Autodesk Fusion 360 part; units mm, degrees
(part 2 of 2)
  constraint tangent L241 A239
  constraint tangent L240 A239
  constraint tangent L231 A240
  constraint tangent L232 A240
  constraint tangent L230 A241
  constraint tangent L231 A241
  constraint tangent L229 A242
  constraint tangent L230 A242
  constraint tangent L228 A243
  constraint tangent L229 A243
  constraint tangent L227 A244
  constraint tangent L228 A244
  constraint tangent L226 A245
  constraint tangent L227 A245
  constraint tangent L226 A246
  constraint tangent L245 A246
  constraint tangent L244 A247
  constraint tangent L245 A247
  constraint tangent L244 A248
  constraint tangent L243 A248
  constraint tangent L242 A249
  constraint tangent L243 A249
  constraint tangent L246 A250
  constraint tangent L240 A250
  constraint tangent L239 A251
  constraint tangent L246 A251
  constraint tangent L247 A252
  constraint tangent L239 A252
  constraint tangent L238 A253
  constraint tangent L247 A253
  constraint tangent L238 A254
  constraint tangent L237 A254
  constraint tangent L237 A255
  constraint tangent L236 A255
  constraint tangent L236 A256
  constraint tangent L235 A256
  constraint tangent L235 A257
  constraint tangent L234 A257
  constraint perpendicular L249 L253
  constraint collinear L251 L252
  constraint collinear L253 L254
  constraint tangent L249 A258
  constraint tangent L251 A258
  constraint tangent L249 A259
  constraint tangent L254 A259
  constraint tangent L250 A260
  constraint tangent L252 A260
  constraint tangent L250 A261
  constraint tangent L253 A261
  constraint concentric A3 A262
  constraint concentric A4 A263
  constraint concentric A0 A264
  constraint concentric A1 A265
  constraint concentric A111 A266
  constraint concentric A112 A267
  constraint vertical L248
  constraint tangent L255 A268
  constraint tangent L256 A268
  constraint tangent L255 A269
  constraint tangent L256 A270
  constraint coincident L213 L257.end
  constraint tangent L248 A271
  constraint coincident L257.start A271.start
  constraint tangent L248 A272
  measures "d1" diameter of A0
  measures "d2" diameter of A1
  measures "d3" diameter of A2
  measures "d4" diameter of A3
  measures "d5" diameter of A4
  measures "d9" diameter of A111
  measures "d12" diameter of A112
  measures "d367" diameter of A262
  measures "d368" diameter of A263
  measures "d369" diameter of A264
  measures "d370" diameter of A265
  measures "d393" diameter of A266
  measures "d394" diameter of A267
extrude "Extrude1" add sketch "mriya" along normal blind 10.5 contours L178 L179 L204 A214 L205 A215 L206 A216 L207 A217 L208 A218 L209 A219 L210 A220 L211 A221 L212 A222 L213 L214 A224 L215 A225 L216 A226 L217 A227 L218 A228 L219 A229 L220 A230 L221 A231 L222 A232 L223 A233 L224 A234 L225 A235 L226 L227 L228 L229 L230 L231 L232 L233 L234 L235 L236 L237 L238 L239 L240 L241 L242 L243 L244 L245 L246 L247 A236 A237 A239 A240 A241 A242 A243 A244 A245 A246 A247 A248 A249 A250 A251 A252 A253 A254 A255 A256 A257 L257 makes body 1
extrude "Extrude2" add sketch "mriya" along normal blind 17 contours L178 L179 L213 A223 L214 L241 L242 A238 bodies 1
extrude "Extrude3" add sketch "mriya" along normal blind 3.7 contours A114 | A115 | A116 | A117 | L204 A214 L205 A215 L206 A216 L207 A217 L208 A218 L209 A219 L210 A220 L211 A221 L212 A222 L213 L214 A224 L215 A225 L216 A226 L217 A227 L218 A228 L219 A229 L220 A230 L221 A231 L222 A232 L223 A233 L224 A234 L225 A235 L248 L255 L256 A268 A269 A270 L257 A271 A272 | L213 A223 L214 L255 L256 A268 A269 A270 | L213 L248 A271 A272 | A266 | A267 bodies 1
extrude "Extrude13" add sketch "mriya" along normal blind 1.8 contours A2 | L108 L109 A118 A119 A120 L186 L187 L190 A198 A199 | A121 L110 A122 L111 A123 L180 L181 L184 A202 A203 | A124 L112 A125 L113 A126 L114 A127 L115 | A128 L116 A129 L117 A130 L118 A131 L119 | A132 L120 A133 A134 L121 L188 L189 L191 A200 A201 | A135 L122 A136 A137 L123 L182 L183 L185 A204 A205 | A138 L124 A139 L125 A140 L126 A141 L127 | A142 L128 A143 L129 A144 L130 A145 L131 | A146 L132 A147 L133 A148 L134 A149 L135 | A150 L136 A151 L137 A152 L138 A153 L139 | A154 L140 A155 L141 A156 L142 A157 L143 | A158 L144 A159 L145 A160 L146 A161 L147 | A162 L148 A163 L149 A164 L150 A165 L151 | A166 L152 A167 L153 A168 L194 L195 L196 A206 A207 | A169 L154 A170 L155 A171 L156 A172 L157 | A173 L158 A174 L159 A175 L200 L201 L202 A210 A211 | A176 L160 A177 L161 A178 L162 A179 L163 | A180 A181 L164 A182 L165 L198 L199 L203 A212 A213 | A183 L166 A184 L167 A185 L168 A186 L169 | A187 A188 L170 A189 L171 L192 L193 L197 A208 A209 | A190 L172 A191 L173 A192 L174 A193 L175 | A194 L176 A195 L249 L251 L254 A258 A259 | A196 L177 A197 L250 L252 L253 A260 A261 bodies 1
extrude "Extrude14" add sketch "mriya" along normal blind 2.2 contours A0 | A1 | A3 | A4 bodies 1
extrude "Extrude6" add sketch "mriya" along normal blind 1 from surface at 14.3 contours L213 A223 L214 L255 L256 A268 A269 A270 bodies 1
extrude "Extrude12" add sketch "mriya" along normal blind 1 from surface at 7.7 contours L213 L248 A271 A272 bodies 1
sketch "power switch" plane through (-4.4, 0, 0) normal (1, 0, 0) x (0, 1, 0)
  line L0 (1.7932, 0) -> (76.6932, 0)
  line L1 (76.6932, 0) -> (76.6932, 17)
  line L2 (76.6932, 17) -> (19.2932, 17)
  line L3 (19.2932, 17) -> (19.2932, 10.5)
  line L4 (19.2932, 10.5) -> (1.7932, 10.5)
  line L5 (1.7932, 10.5) -> (1.7932, 0)
  line L6 (24.0932, 4.15) -> (24.0932, 9.1)
  line L7 (37.2932, 3.75) -> (24.4932, 3.75)
  arc A0 (37.6932, 9.1) -> (37.2932, 9.5) centre (37.2932, 9.1) ccw
  line L8 (36.0932, 8.1) -> (36.0932, 5.15)
  line L9 (25.6932, 8.1) -> (36.0932, 8.1)
  line L10 (36.0932, 5.15) -> (25.6932, 5.15)
  line L11 (25.6932, 5.15) -> (25.6932, 8.1)
  line L12 (24.4932, 9.5) -> (37.2932, 9.5)
  arc A1 (24.0932, 4.15) -> (24.4932, 3.75) centre (24.4932, 4.15) ccw
  arc A2 (37.2932, 3.75) -> (37.6932, 4.15) centre (37.2932, 4.15) ccw
  line L13 (37.6932, 9.1) -> (37.6932, 4.15)
  arc A3 (24.4932, 9.5) -> (24.0932, 9.1) centre (24.4932, 9.1) ccw
  constraint perpendicular L10 L11
  constraint vertical L11
  constraint perpendicular L9 L11
  constraint vertical L8
  constraint tangent A0 L12
  constraint tangent A0 L13
  constraint tangent A2 L13
  constraint tangent L7 A2
  constraint tangent L7 A1
  constraint tangent L6 A1
  constraint tangent L6 A3
  constraint tangent L12 A3
extrude "Extrude8" cut sketch "power switch" against normal blind 2.5 contours L8 L9 L10 L11 bodies 1
extrude "Extrude9" cut sketch "power switch" against normal blind 1 contours L6 L7 A0 L12 A1 A2 L13 A3 bodies 1
chamfer "Chamfer13" distance 1.19 angle 40 8 edges at (-4.4, 30.8932, 3.75) (-4.4, 24.2104, 3.8672) (-4.4, 24.0932, 6.625) (-4.4, 24.2104, 9.3828) (-4.4, 30.8932, 9.5) (-4.4, 37.576, 9.3828) (-4.4, 37.6932, 6.625) (-4.4, 37.576, 3.8672) measured on face at (-4.4, 63.6932, 8.7) measured on face at (-4.4, 63.6932, 8.7) measured on face at (-4.4, 63.6932, 8.7) measured on face at (-4.4, 63.6932, 8.7) measured on face at (-4.4, 63.6932, 8.7) measured on face at (-4.4, 63.6932, 8.7) measured on face at (-4.4, 63.6932, 8.7) measured on face at (-4.4, 63.6932, 8.7) on bodies 1
chamfer "Chamfer14" distance 0.8 angle 45 4 edges at (-6.9, 30.8932, 5.15) (-6.9, 25.6932, 6.625) (-6.9, 30.8932, 8.1) (-6.9, 36.0932, 6.625) on bodies 1
sketch "usb-c" plane through (0, 80.6932, 0) normal (0, 1, 0) x (-1, 0, 0)
  line L0 (8.4, 0) -> (41.0674, 0)
  line L1 (41.0674, 0) -> (41.0674, 10.5)
  line L2 (41.0674, 10.5) -> (25.8, 10.5)
  line L3 (25.8, 10.5) -> (25.8, 17)
  line L4 (25.8, 17) -> (8.4, 17)
  line L5 (8.4, 17) -> (8.4, 0)
  line L6 (19.7003, 8.8) -> (13.1003, 8.8)
  line L7 (21.9003, 12.8) -> (21.9003, 8.4)
  line L8 (21.1002, 11) -> (21.1002, 10.2)
  arc A0 (11.3003, 13.2) -> (10.9002, 12.8) centre (11.3003, 12.8) ccw
  arc A1 (21.5003, 8) -> (21.9002, 8.4) centre (21.5003, 8.4) ccw
  arc A2 (19.7003, 8.8) -> (21.1003, 10.2) centre (19.7003, 10.2) ccw
  line L9 (11.7003, 10.2) -> (11.7003, 11)
  line L10 (21.5003, 8) -> (11.3002, 8)
  arc A3 (21.1002, 11) -> (19.7003, 12.4) centre (19.7003, 11) ccw
  arc A4 (13.1002, 12.4) -> (11.7002, 11) centre (13.1002, 11) ccw
  line L11 (11.3003, 13.2) -> (21.5003, 13.2)
  line L12 (13.1002, 12.4) -> (19.7003, 12.4)
  arc A5 (21.9002, 12.8) -> (21.5003, 13.2) centre (21.5003, 12.8) ccw
  arc A6 (10.9002, 8.4) -> (11.3002, 8) centre (11.3002, 8.4) ccw
  line L13 (10.9002, 8.4) -> (10.9002, 12.8)
  arc A7 (11.7003, 10.2) -> (13.1003, 8.8) centre (13.1003, 10.2) ccw
  constraint tangent L9 A4
  constraint tangent A4 L12
  constraint tangent A3 L12
  constraint tangent L8 A3
  constraint tangent L6 A2
  constraint tangent L8 A2
  constraint tangent L6 A7
  constraint tangent L9 A7
  constraint perpendicular L7 L11
  constraint perpendicular L10 L13
  constraint horizontal L10
  constraint perpendicular L7 L10
  constraint tangent A0 L11
  constraint tangent A0 L13
  constraint tangent L11 A5
  constraint tangent L7 A5
  constraint tangent A6 L13
  constraint tangent L10 A6
  constraint tangent A1 L10
  constraint tangent L7 A1
extrude "Extrude17" cut sketch "usb-c" against normal blind 2.5 contours L6 L8 A2 L9 A3 A4 L12 A7 bodies 1
extrude "Extrude18" cut sketch "usb-c" against normal blind 1 contours L7 A0 A1 L10 L11 A5 A6 L13 bodies 1
chamfer "Chamfer23" distance 1.19 angle 40 8 edges at (-16.4003, 80.6932, 8) (-11.0174, 80.6932, 8.1172) (-10.9003, 80.6932, 10.6) (-11.0174, 80.6932, 13.0828) (-16.4003, 80.6932, 13.2) (-21.7831, 80.6932, 13.0828) (-21.9003, 80.6932, 10.6) (-21.7831, 80.6932, 8.1172) measured on face at (-23.679, 80.6932, 2.6687) measured on face at (-23.679, 80.6932, 2.6687) measured on face at (-23.679, 80.6932, 2.6687) measured on face at (-23.679, 80.6932, 2.6687) measured on face at (-23.679, 80.6932, 2.6687) measured on face at (-23.679, 80.6932, 2.6687) measured on face at (-23.679, 80.6932, 2.6687) measured on face at (-23.679, 80.6932, 2.6687) on bodies 1
chamfer "Chamfer21" distance 0.599 angle 45 3 edges at (-14.85, 78.1932, 14.3) (-7.3979, 77.6953, 14.3) (-6.9, 57.7432, 14.3) on bodies 1
chamfer "Chamfer22" distance 0.6 angle 45 1 edges at (-6.9, 9.5932, 7.7) on bodies 1
chamfer "Chamfer17" distance 1 angle 45 90 edges at (-17.0879, -2.2068, 10.5) (-5.5716, -1.0352, 10.5) (-4.4, 10.5432, 10.5) (-33.4337, 80.6932, 10.5) (-41.4501, 80.7693, 10.5) (-42.3387, 81.5503, 10.5) (-43.8762, 82.7648, 10.5) (-51.4458, 82.9932, 10.5) (-58.2501, 83.0693, 10.5) (-60.2387, 84.9503, 10.5) (-62.8762, 87.2648, 10.5) (-73.4, 87.4932, 10.5) (-83.9238, 87.2648, 10.5) (-86.0613, 85.4503, 10.5) (-87.5499, 84.0693, 10.5) (-94.8542, 83.9932, 10.5) (-102.9238, 83.7648, 10.5) (-107.238, 79.7735, 10.5) (-111.0657, 76.1074, 10.5) (-116.2077, 75.9932, 10.5) (-121.9238, 75.7648, 10.5) (-123.4613, 74.5503, 10.5) (-124.3499, 73.7693, 10.5) (-131.5163, 73.6932, 10.5) (-141.1284, 72.5216, 10.5) (-142.3, 42.8932, 10.5) (-141.1284, 13.2648, 10.5) (-120.4728, 12.0932, 10.5) (-100.9235, 12.4357, 10.5) (-96.4155, 16.4593, 10.5) (-92.7186, 19.941, 10.5) (-84.5898, 20.0932, 10.5) (-75.7143, 19.6842, 10.5) (-70.5474, 11.3702, 10.5) (-65.1972, 2.8703, 10.5) (-56.0828, 2.3932, 10.5) (-48.3499, 2.3171, 10.5) (-47.4613, 1.5361, 10.5) (-45.9238, 0.3216, 10.5) (-37.2542, 0.0932, 10.5) (-29.3499, 0.0171, 10.5) (-28.4613, -0.7639, 10.5) (-26.9238, -1.9784, 10.5) (-17.0879, -2.2068, 0) (-26.9238, -1.9784, 0) (-28.4613, -0.7639, 0) (-29.3499, 0.0171, 0) (-37.2542, 0.0932, 0) (-45.9238, 0.3216, 0) (-47.4613, 1.5361, 0) (-48.3499, 2.3171, 0) (-56.0828, 2.3932, 0) (-65.1972, 2.8703, 0) (-70.5474, 11.3702, 0) (-75.7143, 19.6842, 0) (-84.5898, 20.0932, 0) (-92.7186, 19.941, 0) (-96.4155, 16.4593, 0) (-100.9235, 12.4357, 0) (-120.4728, 12.0932, 0) (-141.1284, 13.2648, 0) (-142.3, 42.8932, 0) (-141.1284, 72.5216, 0) (-131.5163, 73.6932, 0) (-124.3499, 73.7693, 0) (-123.4613, 74.5503, 0) (-121.9238, 75.7648, 0) (-116.2077, 75.9932, 0) (-111.0657, 76.1074, 0) (-107.238, 79.7735, 0) (-102.9238, 83.7648, 0) (-94.8542, 83.9932, 0) (-87.5499, 84.0693, 0) (-86.0613, 85.4503, 0) (-83.9238, 87.2648, 0) (-73.4, 87.4932, 0) (-62.8762, 87.2648, 0) (-60.2387, 84.9503, 0) (-58.2501, 83.0693, 0) (-51.4458, 82.9932, 0) (-43.8762, 82.7648, 0) (-42.3387, 81.5503, 0) (-41.4501, 80.7693, 0) (-24.7337, 80.6932, 0) (-5.5716, 79.5216, 0) (-4.4, 39.2432, 0) (-5.5716, -1.0352, 0) (-4.4, 47.9932, 17) (-5.5716, 79.5216, 17) (-17.1, 80.6932, 17) on bodies 1
fillet "Fillet29" radius 1.2 2 edges at (-4.4, 19.2932, 12.75) (-25.8, 80.6932, 12.75) on bodies 1
chamfer "Chamfer18" distance 1 angle 45 4 edges at (-6.25, 19.2932, 17) (-5.4996, 19.2974, 17) (-25.8, 78.8432, 17) (-25.7958, 79.5936, 17) on bodies 1
chamfer "Chamfer20" distance 0.9 angle 45 6 edges at (-11.1256, 22.891, 0) (-23.6256, 22.891, 0) (-45.9256, 22.941, 0) (-45.9256, 60.941, 0) (-121.9256, 34.941, 0) (-121.9256, 53.941, 0) on bodies 1
sketch "silicone feets" plane through (0, 0, 0) normal (0, 0, -1) x (1, 0, 0)
  circle A0 centre (-120.9, -34.5432) radius 2
  circle A1 centre (-44.9, -22.5432) radius 2
  circle A2 centre (-10.1, -22.4932) radius 2
  line L0 (-8.4, 1.2068) -> (-25.7757, 1.2068)
  arc A3 (-25.7757, 1.2068) -> (-27.1899, 0.621) centre (-25.7757, -0.7932) ccw
  line L1 (-27.1899, 0.621) -> (-28.3184, -0.5074)
  arc A4 (-29.7326, -1.0932) -> (-28.3184, -0.5074) centre (-29.7326, 0.9068) ccw
  line L2 (-29.7326, -1.0932) -> (-44.7757, -1.0932)
  arc A5 (-44.7757, -1.0932) -> (-46.1899, -1.679) centre (-44.7757, -3.0932) ccw
  line L3 (-46.1899, -1.679) -> (-47.3184, -2.8074)
  arc A6 (-48.7326, -3.3932) -> (-47.3184, -2.8074) centre (-48.7326, -1.3932) ccw
  line L4 (-48.7326, -3.3932) -> (-63.4331, -3.3932)
  arc A7 (-63.4331, -3.3932) -> (-65.6097, -4.6635) centre (-63.4331, -5.8932) ccw
  line L5 (-65.6097, -4.6635) -> (-73.7438, -19.0608)
  arc A8 (-77.2264, -21.0932) -> (-73.7438, -19.0608) centre (-77.2264, -17.0932) ccw
  line L6 (-77.2264, -21.0932) -> (-91.9532, -21.0932)
  arc A9 (-94.0745, -20.2145) -> (-91.9532, -21.0932) centre (-91.9532, -18.0932) ccw
  line L7 (-94.0745, -20.2145) -> (-100.1707, -14.1183)
  arc A10 (-100.1707, -14.1183) -> (-102.6456, -13.0932) centre (-102.6456, -16.5932) ccw
  line L8 (-102.6456, -13.0932) -> (-138.3, -13.0932)
  arc A11 (-138.3, -13.0932) -> (-141.3, -16.0932) centre (-138.3, -16.0932) ccw
  line L9 (-141.3, -16.0932) -> (-141.3, -69.6932)
  arc A12 (-141.3, -69.6932) -> (-138.3, -72.6932) centre (-138.3, -69.6932) ccw
  line L10 (-138.3, -72.6932) -> (-124.7326, -72.6932)
  arc A13 (-123.3184, -73.279) -> (-124.7326, -72.6932) centre (-124.7326, -74.6932) ccw
  line L11 (-123.3184, -73.279) -> (-122.1899, -74.4074)
  arc A14 (-122.1899, -74.4074) -> (-120.7757, -74.9932) centre (-120.7757, -72.9932) ccw
  line L12 (-120.7757, -74.9932) -> (-111.6397, -74.9932)
  arc A15 (-109.8719, -75.7254) -> (-111.6397, -74.9932) centre (-111.6397, -77.4932) ccw
  line L13 (-109.8719, -75.7254) -> (-103.19, -82.4074)
  arc A16 (-103.19, -82.4074) -> (-101.7757, -82.9932) centre (-101.7757, -80.9932) ccw
  line L14 (-101.7757, -82.9932) -> (-87.9326, -82.9932)
  arc A17 (-86.5184, -83.579) -> (-87.9326, -82.9932) centre (-87.9326, -84.9932) ccw
  line L15 (-86.5184, -83.579) -> (-84.19, -85.9074)
  arc A18 (-84.19, -85.9074) -> (-82.7757, -86.4932) centre (-82.7757, -84.4932) ccw
  line L16 (-82.7757, -86.4932) -> (-64.0243, -86.4932)
  arc A19 (-64.0243, -86.4932) -> (-62.6101, -85.9074) centre (-64.0243, -84.4932) ccw
  line L17 (-62.6101, -85.9074) -> (-59.2816, -82.579)
  arc A20 (-57.8674, -81.9932) -> (-59.2816, -82.579) centre (-57.8674, -83.9932) ccw
  line L18 (-57.8674, -81.9932) -> (-45.0243, -81.9932)
  arc A21 (-45.0243, -81.9932) -> (-43.6101, -81.4074) centre (-45.0243, -79.9932) ccw
  line L19 (-43.6101, -81.4074) -> (-42.4816, -80.279)
  arc A22 (-41.0674, -79.6932) -> (-42.4816, -80.279) centre (-41.0674, -81.6932) ccw
  line L20 (-41.0674, -79.6932) -> (-8.4, -79.6932)
  arc A23 (-8.4, -79.6932) -> (-5.4, -76.6932) centre (-8.4, -76.6932) ccw
  line L21 (-5.4, -76.6932) -> (-5.4, -1.7932)
  arc A24 (-5.4, -1.7932) -> (-8.4, 1.2068) centre (-8.4, -1.7932) ccw
  circle A25 centre (-22.6, -22.4932) radius 2
  circle A26 centre (-44.9, -60.5432) radius 2
  circle A27 centre (-120.9, -53.5432) radius 2
  circle A28 centre (-10.9, -74.1932) radius 4
  circle A29 centre (-73.4, -80.9932) radius 4
  circle A30 centre (-135.8, -67.1932) radius 4
  circle A31 centre (-135.8, -18.5932) radius 4
  circle A32 centre (-61.6823, -8.8932) radius 4
  circle A33 centre (-10.9, -4.2932) radius 4
  dimension "d374" = 8
  dimension "d375" = 8
  dimension "d376" = 8
  dimension "d377" = 8
  dimension "d378" = 8
  dimension "d379" = 8
  dimension "d380" = 5.5
  dimension "d381" = 5.5
  dimension "d382" = 5.5
  dimension "d383" = 5.5
  dimension "d384" = 5.5
  dimension "d385" = 5.5
  dimension "d386" = 5.5
  dimension "d387" = 5.5
  dimension "d388" = 5.5
  dimension "d389" = 5.5
  dimension "d390" = 5.5
  measures "d374" diameter of A28
  measures "d375" diameter of A29
  measures "d376" diameter of A30
  measures "d377" diameter of A31
  measures "d378" diameter of A32
  measures "d379" diameter of A33
  measures "d380" distance of L20 A28.centre
  measures "d381" distance of L21 A28.centre
  measures "d382" distance of L16 A29.centre
  measures "d383" distance of L10 A30.centre
  measures "d384" distance of L9 A30.centre
  measures "d385" distance of L9 A31.centre
  measures "d386" distance of L8 A31.centre
  measures "d387" distance of L5 A32.centre
  measures "d388" distance of L4 A32.centre
  measures "d389" distance of L0 A33.centre
  measures "d390" distance of L21 A33.centre
extrude "Extrude15" cut sketch "silicone feets" against normal blind 0.8 contours A28 | A29 | A30 | A31 | A32 | A33 bodies 1
extrude "Extrude16" cut sketch "mriya" along normal blind 1 from surface at 2.7 contours A266 | A267 bodies 1
mirror "Mirror1" about plane through (0, 0, 0) normal (1, 0, 0) of bodies 1 makes body 2
named bodies: "Left", "Right"
